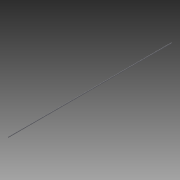
# Autodesk Inventor part: vee-track
Saved by Autodesk Inventor 2013 (Build 170138000, 138)
## iProperties
Created: 2012-11-27
Part Number: vee-track
Material: Generic
Document SubType Name: Modeling
Designer: istvan.burbank
Density: 1 g/cm^3
Author: istvan.burbank
Autodesk Inventor part; units mm, degrees
ref_plane "YZ Plane" through (0, 0, 0) normal (1, 0, 0) x (0, 1, 0)
ref_plane "XZ Plane" through (0, 0, 0) normal (0, 1, 0) x (-1, 0, 0)
ref_plane "Work Plane1" through (-1.2283, 0, 317.5) normal (0, 0, 1) x (1, 0, 0)
sketch "Sketch1" plane through (-1.2283, 0, 317.5) normal (0, 0, 1) x (1, 0, 0)
  line L0 (-0.3592, 8.7122) -> (-0.3592, 0.3592) projected
  line L1 (-0.3592, 0.3592) -> (0, 0) projected
  line L2 (0, 0) -> (2.4566, 0) projected
  line L3 (2.4566, 0) -> (2.8158, 0.3592) projected
  line L4 (2.8158, 0.3592) -> (2.8158, 7.6708) projected
  line L5 (2.8158, 7.6708) -> (2.6888, 7.6708) projected
  arc A0 (2.6888, 7.9248) -> (2.6888, 7.6708) centre (2.6888, 7.7978) ccw projected
  line L6 (2.6888, 7.9248) -> (4.3906, 7.9248) projected
  line L7 (4.3906, 7.9248) -> (4.3906, 8.7376) projected
  line L8 (4.3906, 8.7376) -> (2.2824, 10.8458) projected
  line L9 (2.2824, 10.8458) -> (1.7744, 10.8458) projected
  line L10 (1.7744, 10.8458) -> (-0.3592, 8.7122) projected
  point P0 (1.2283, 0)
extrude "Extrusion1" add sketch "Sketch1" against normal blind 1828.8
body "Solid2"
